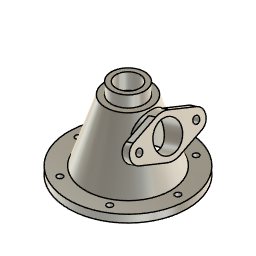
exercise07 (Autodesk Fusion 360 design; units mm, degrees)
Autodesk Fusion 360 part; units mm, degrees
sketch "草图1" plane through (0, 0, 0) normal (0, 1, 0) x (1, 0, 0)
  line L0 (0, -80) -> (0, 30) construction
  line L1 (42.368, 0) -> (62.5, 0)
  line L2 (62.5, 0) -> (62.5, -8)
  line L3 (62.5, -8) -> (45, -8)
  line L4 (45, -8) -> (23.6189, -73)
  line L5 (23.6189, -73) -> (17.5, -73)
  line L6 (17.5, -73) -> (17.5, -85)
  line L7 (17.5, -85) -> (12.5, -85)
  line L8 (12.5, -85) -> (12.5, -68)
  line L9 (12.5, -68) -> (20, -68)
  line L10 (20, -68) -> (42.368, 0)
  dimension "d1" = 5
  dimension "d2" = 8
  dimension "d3" = 62.5
  dimension "d4" = 45
  dimension "d5" = 5
  dimension "d7" = 12
  dimension "d8" = 5
  dimension "d9" = 17.5
  dimension "d10" = 20
  dimension "d11" = 85
  constraint perpendicular L0 L1
  constraint perpendicular L1 L2
  constraint perpendicular L2 L3
  constraint perpendicular L2 L5
  constraint perpendicular L5 L6
  constraint perpendicular L6 L7
  constraint perpendicular L7 L8
  constraint perpendicular L8 L9
  constraint parallel L4 L10
  constraint collinear origin L1.start L1.end
  measures "d1" distance of L6.end L7.end
  measures "d2" distance of L1.end L2.end
  measures "d3" distance of origin L1.end
  measures "d4" distance of L0 L3.end
  measures "d5" distance of L4 L10
  measures "d7" distance of L5.end L6.end
  measures "d8" distance of L5 L9
  measures "d9" distance of L0 L6.end
  measures "d10" distance of L0 L9.end
  measures "d11" distance of L1 L7
revolve "旋转1" add sketch "草图1" angle 360 about axis through (0, 0, 80) along (0, 0, -1) makes body 1
sketch "草图2" plane through (0, 0, 8) normal (0, 0, 1) x (-1, 0, 0)
  circle A0 centre (0, 0) radius 62.5
  circle A1 centre (0, 0) radius 45
  circle A2 centre (-52.5, 0) radius 3
  circle A3 centre (-26.25, -45.4663) radius 3
  circle A4 centre (26.25, -45.4663) radius 3
  circle A5 centre (52.5, 0) radius 3
  circle A6 centre (26.25, 45.4663) radius 3
  circle A7 centre (-26.25, 45.4663) radius 3
  dimension "d13" = 6
  dimension "d14" = 52.5
  dimension "d16" = 360
  measures "d13" diameter of A2
  measures "d14" distance of A0.centre A2.centre
extrude "拉伸1" cut sketch "草图2" against normal blind 20 contours A2 | A3 | A4 | A5 | A6 | A7 bodies 1
sketch "草图3" plane through (0, 0, 0) normal (0, 1, 0) x (1, 0, 0)
ref_plane "工作平面1" through (34.3094, 0, 40.5) normal (0.949928, 0, 0.31247) x (0, -1, 0)
ref_plane "工作平面2" through (45.7086, 0, 44.2496) normal (0.949928, 0, 0.31247) x (0, -1, 0)
sketch "草图4" plane through (54.38, 0, 17.8878) normal (0.949928, 0, 0.31247) x (0, -1, 0)
sketch "草图5" plane through (54.38, 0, 17.8878) normal (0.949928, 0, 0.31247) x (0, -1, 0)
  circle A0 centre (-30, -40) radius 3.5
  circle A1 centre (30, -40) radius 3.5
  line L0 (33.3333, -49.4281) -> (6.6667, -58.8562)
  line L1 (33.3333, -30.5719) -> (6.6667, -21.1438)
  line L2 (-33.3333, -30.5719) -> (-6.6667, -21.1438)
  line L3 (-33.3333, -49.4281) -> (-6.6667, -58.8562)
  circle A2 centre (0, -40) radius 15
  line L4 (0, -75) -> (0, 0) construction
  arc A3 (33.3333, -49.4281) -> (33.3333, -30.5719) centre (30, -40) ccw
  arc A4 (6.6667, -21.1438) -> (-6.6667, -21.1438) centre (0, -40) ccw
  arc A5 (-6.6667, -58.8562) -> (6.6667, -58.8562) centre (0, -40) ccw
  arc A6 (-33.3333, -30.5719) -> (-33.3333, -49.4281) centre (-30, -40) ccw
  line L5 (0, 13.2387) -> (0, 19.5294)
  point P0 (0, -75.9942)
  dimension "d21" = 7
  dimension "d22" = 20
  dimension "d23" = 40
  dimension "d24" = 60
  dimension "d25" = 30
  dimension "d27" = 30
  dimension "d29" = 50
  constraint concentric A0 A6
  constraint concentric A1 A3
  constraint coincident L3.end A4
  constraint equal A3 A6
  constraint equal A0 A1
  constraint concentric A2 A4
  constraint coincident L4.end origin
  constraint vertical L4
  constraint symmetric A0.centre A1.centre L4
  constraint collinear L4.end A2.centre P0
  constraint collinear A2.centre A0.centre A1.centre
  constraint tangent L3 A6
  constraint tangent L2 A4
  constraint tangent L2 A6
  constraint tangent L1 A4
  constraint tangent L1 A3
  constraint tangent L0 A3
  constraint tangent L0 A4
  constraint coincident L3 A5.start
  constraint concentric A4 A5
  constraint symmetric L0 L3 L4
  constraint equal A4 A5
  measures "d21" diameter of A0
  measures "d22" diameter of A6
  measures "d23" diameter of A4
  measures "d24" horizontal distance of A0.centre A1.centre
  measures "d25" diameter of A2
  measures "d27" distance of A1.centre L5
  measures "d29" distance of A1.centre L4.end
extrude "拉伸2" add sketch "草图5" against normal blind 8 separate body makes body 2
sketch "草图6" plane through (54.38, 0, 17.8878) normal (0.949928, 0, 0.31247) x (0, 1, 0)
  circle A0 centre (30, 40) radius 3.5
  circle A1 centre (-30, 40) radius 3.5
  circle A2 centre (0, 40) radius 15
  arc A3 (-33.3333, 49.4281) -> (-33.3333, 30.5719) centre (-30, 40) ccw
  line L0 (-33.3333, 30.5719) -> (-6.6667, 21.1438)
  arc A4 (-6.6667, 21.1438) -> (6.6667, 21.1438) centre (0, 40) ccw
  line L1 (6.6667, 21.1438) -> (33.3333, 30.5719)
  arc A5 (33.3333, 30.5719) -> (33.3333, 49.4281) centre (30, 40) ccw
  line L2 (33.3333, 49.4281) -> (6.6667, 58.8562)
  arc A6 (6.6667, 58.8562) -> (-6.6667, 58.8562) centre (0, 40) ccw
  line L3 (-6.6667, 58.8562) -> (-33.3333, 49.4281)
  circle A7 centre (0, 40) radius 20
  circle A8 centre (0, 40) radius 15
  constraint concentric A2 A7
  constraint concentric A7 A8
extrude "拉伸3" add sketch "草图6" along normal up to surface contours A4 A6 A7 end surface at (-14.1168, 35.9689, 11.3333) on bodies 1 bodies 1 2
extrude "拉伸4" cut sketch "草图6" along normal up to surface contours A2 A8 end surface at (35.1613, -4.3771, 21.0837) on bodies 1 bodies 1
equation "d3 = ( 125 / 2 ) * 1 mm"
equation "d14 = ( 105 / 2 ) * 1 mm"
